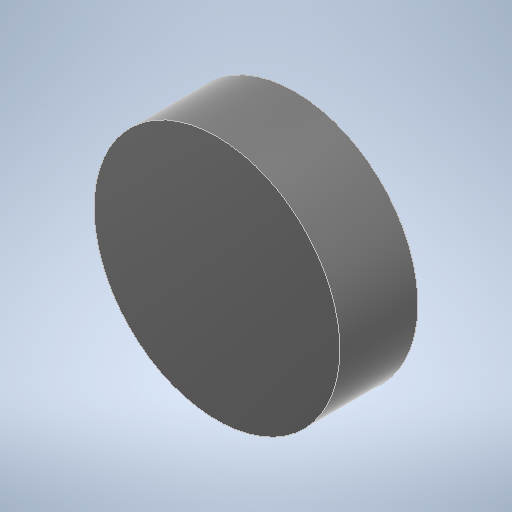
# Autodesk Inventor part: Spring_Top
Saved by Autodesk Inventor 2025.1 (Build 291241020, 241B)
## iProperties
Created: 2024-11-13
Part Number: Spring_Top
Material: PC/ABS Plastic
Document SubType Name: Modeling
Designer: leon-
Density: 1.1 g/cm^3
Appearance: Smooth - Black
Author: leon-
Autodesk Inventor part; units mm, degrees
ref_plane "YZ Plane" through (0, 0, 0) normal (1, 0, 0) x (0, 1, 0)
ref_plane "XZ Plane" through (0, 0, 0) normal (0, 1, 0) x (-1, 0, 0)
ref_plane "XY Plane" through (0, 0, 0) normal (0, 0, 1) x (1, 0, 0)
sketch "Sketch1" plane through (0, 0, 0) normal (1, 0, 0) x (0, 1, 0)
  line L0 (0, 0) -> (15.75, 0)
  line L1 (15.75, 0) -> (15.75, -10)
  line L2 (15.75, -10) -> (10.2, -10)
  line L3 (10.2, -10) -> (10.2, -5)
  line L4 (10.2, -5) -> (0, -5)
  line L5 (0, -5) -> (0, 0)
  point P0 (0, -2.5)
  point P1 (15.75, -5)
  point P2 (7.875, 0)
  dimension "d0" = 15.75
  dimension "d1" = 10.2
  dimension "d2" = 10
  dimension "d3" = 5
  constraints: 12 end point, 5 perpendicular, 3 midpoint, 1 horizontal
  measures "d0" horizontal distance of point (0, -2.5) point (15.75, -5)
  measures "d1" distance between parallel lines of L5 L3
  measures "d2" distance between parallel lines of L0 L2
  measures "d3" distance from line of point (7.875, 0) L4
revolve "Revolution1" add sketch "Sketch1" angle 360 about axis through (0, 0, -5) along (0, 0, 1)
body "Solid1"
